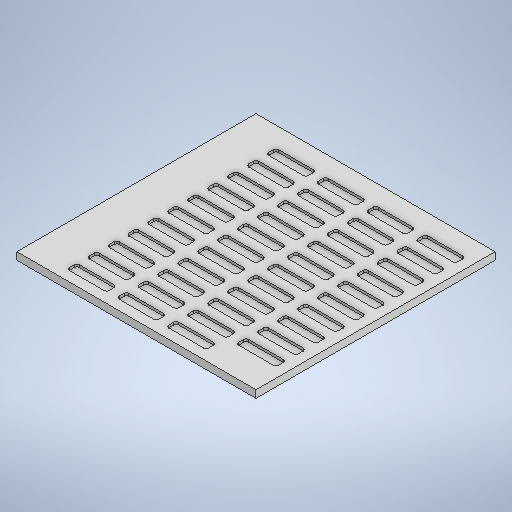
# Autodesk Inventor part: mold plate
Saved by Autodesk Inventor 2025.3 (Build 293356030, 356C)
## iProperties
Created: 2025-07-29
Part Number: mold plate
Material: Generic
Document SubType Name: Modeling
Designer: toppe
Density: 1 g/cm^3
Appearance: Default
Author: toppe
Autodesk Inventor part; units mm, degrees
ref_plane "YZ Plane" through (0, 0, 0) normal (1, 0, 0) x (0, 1, 0)
ref_plane "XZ Plane" through (0, 0, 0) normal (0, 1, 0) x (-1, 0, 0)
ref_plane "XY Plane" through (0, 0, 0) normal (0, 0, 1) x (1, 0, 0)
sketch "Sketch1" plane through (0, 0, 0) normal (0, 1, 0) x (-1, 0, 0)
  line L0 (0, 0) -> (304.8, 0)
  line L1 (304.8, 0) -> (304.8, -304.8)
  line L2 (304.8, -304.8) -> (0, -304.8)
  line L3 (0, -304.8) -> (0, 0)
  dimension "d0" = 304.8
  dimension "d1" = 304.8
  constraints: 8 end point, 2 parallel, 1 horizontal, 1 perpendicular
  measures "d0" distance of L0.end L1.end
  measures "d1" distance of L0.start L0.end
extrude "Extrusion1" add sketch "Sketch1" along normal blind 9.525
sketch "Sketch2" plane through (0, 9.525, 0) normal (0, 1, 0) x (1, 0, 0)
  line L0 (-60.325, 12.7) -> (-15.875, 12.7)
  line L1 (-12.7, 15.875) -> (-12.7, 22.225)
  line L2 (-15.875, 25.4) -> (-60.325, 25.4)
  line L3 (-63.5, 22.225) -> (-63.5, 15.875)
  line L4 (-304.8, 0) -> (0, 0) projected
  line L5 (0, 0) -> (0, 304.8) projected
  arc A0 (-63.5, 15.875) -> (-60.325, 12.7) centre (-60.325, 15.875) ccw
  arc A1 (-60.325, 25.4) -> (-63.5, 22.225) centre (-60.325, 22.225) ccw
  arc A2 (-15.875, 12.7) -> (-12.7, 15.875) centre (-15.875, 15.875) ccw
  arc A3 (-12.7, 22.225) -> (-15.875, 25.4) centre (-15.875, 22.225) ccw
  line L6 (-60.325, 38.1) -> (-15.875, 38.1)
  line L7 (-12.7, 41.275) -> (-12.7, 47.625)
  line L8 (-15.875, 50.8) -> (-60.325, 50.8)
  line L9 (-63.5, 47.625) -> (-63.5, 41.275)
  arc A4 (-15.875, 38.1) -> (-12.7, 41.275) centre (-15.875, 41.275) ccw
  arc A5 (-60.325, 50.8) -> (-63.5, 47.625) centre (-60.325, 47.625) ccw
  arc A6 (-63.5, 41.275) -> (-60.325, 38.1) centre (-60.325, 41.275) ccw
  arc A7 (-12.7, 47.625) -> (-15.875, 50.8) centre (-15.875, 47.625) ccw
  line L10 (-60.325, 63.5) -> (-15.875, 63.5)
  line L11 (-12.7, 66.675) -> (-12.7, 73.025)
  line L12 (-15.875, 76.2) -> (-60.325, 76.2)
  line L13 (-63.5, 73.025) -> (-63.5, 66.675)
  arc A8 (-15.875, 63.5) -> (-12.7, 66.675) centre (-15.875, 66.675) ccw
  arc A9 (-60.325, 76.2) -> (-63.5, 73.025) centre (-60.325, 73.025) ccw
  arc A10 (-63.5, 66.675) -> (-60.325, 63.5) centre (-60.325, 66.675) ccw
  arc A11 (-12.7, 73.025) -> (-15.875, 76.2) centre (-15.875, 73.025) ccw
  line L14 (-60.325, 88.9) -> (-15.875, 88.9)
  line L15 (-12.7, 92.075) -> (-12.7, 98.425)
  line L16 (-15.875, 101.6) -> (-60.325, 101.6)
  line L17 (-63.5, 98.425) -> (-63.5, 92.075)
  arc A12 (-15.875, 88.9) -> (-12.7, 92.075) centre (-15.875, 92.075) ccw
  arc A13 (-60.325, 101.6) -> (-63.5, 98.425) centre (-60.325, 98.425) ccw
  arc A14 (-63.5, 92.075) -> (-60.325, 88.9) centre (-60.325, 92.075) ccw
  arc A15 (-12.7, 98.425) -> (-15.875, 101.6) centre (-15.875, 98.425) ccw
  line L18 (-60.325, 114.3) -> (-15.875, 114.3)
  line L19 (-12.7, 117.475) -> (-12.7, 123.825)
  line L20 (-15.875, 127) -> (-60.325, 127)
  line L21 (-63.5, 123.825) -> (-63.5, 117.475)
  arc A16 (-15.875, 114.3) -> (-12.7, 117.475) centre (-15.875, 117.475) ccw
  arc A17 (-60.325, 127) -> (-63.5, 123.825) centre (-60.325, 123.825) ccw
  arc A18 (-63.5, 117.475) -> (-60.325, 114.3) centre (-60.325, 117.475) ccw
  arc A19 (-12.7, 123.825) -> (-15.875, 127) centre (-15.875, 123.825) ccw
  line L22 (-60.325, 139.7) -> (-15.875, 139.7)
  line L23 (-12.7, 142.875) -> (-12.7, 149.225)
  line L24 (-15.875, 152.4) -> (-60.325, 152.4)
  line L25 (-63.5, 149.225) -> (-63.5, 142.875)
  arc A20 (-15.875, 139.7) -> (-12.7, 142.875) centre (-15.875, 142.875) ccw
  arc A21 (-60.325, 152.4) -> (-63.5, 149.225) centre (-60.325, 149.225) ccw
  arc A22 (-63.5, 142.875) -> (-60.325, 139.7) centre (-60.325, 142.875) ccw
  arc A23 (-12.7, 149.225) -> (-15.875, 152.4) centre (-15.875, 149.225) ccw
  line L26 (-60.325, 165.1) -> (-15.875, 165.1)
  line L27 (-12.7, 168.275) -> (-12.7, 174.625)
  line L28 (-15.875, 177.8) -> (-60.325, 177.8)
  line L29 (-63.5, 174.625) -> (-63.5, 168.275)
  arc A24 (-15.875, 165.1) -> (-12.7, 168.275) centre (-15.875, 168.275) ccw
  arc A25 (-60.325, 177.8) -> (-63.5, 174.625) centre (-60.325, 174.625) ccw
  arc A26 (-63.5, 168.275) -> (-60.325, 165.1) centre (-60.325, 168.275) ccw
  arc A27 (-12.7, 174.625) -> (-15.875, 177.8) centre (-15.875, 174.625) ccw
  line L30 (-60.325, 190.5) -> (-15.875, 190.5)
  line L31 (-12.7, 193.675) -> (-12.7, 200.025)
  line L32 (-15.875, 203.2) -> (-60.325, 203.2)
  line L33 (-63.5, 200.025) -> (-63.5, 193.675)
  arc A28 (-15.875, 190.5) -> (-12.7, 193.675) centre (-15.875, 193.675) ccw
  arc A29 (-60.325, 203.2) -> (-63.5, 200.025) centre (-60.325, 200.025) ccw
  arc A30 (-63.5, 193.675) -> (-60.325, 190.5) centre (-60.325, 193.675) ccw
  arc A31 (-12.7, 200.025) -> (-15.875, 203.2) centre (-15.875, 200.025) ccw
  line L34 (-60.325, 215.9) -> (-15.875, 215.9)
  line L35 (-12.7, 219.075) -> (-12.7, 225.425)
  line L36 (-15.875, 228.6) -> (-60.325, 228.6)
  line L37 (-63.5, 225.425) -> (-63.5, 219.075)
  arc A32 (-15.875, 215.9) -> (-12.7, 219.075) centre (-15.875, 219.075) ccw
  arc A33 (-60.325, 228.6) -> (-63.5, 225.425) centre (-60.325, 225.425) ccw
  arc A34 (-63.5, 219.075) -> (-60.325, 215.9) centre (-60.325, 219.075) ccw
  arc A35 (-12.7, 225.425) -> (-15.875, 228.6) centre (-15.875, 225.425) ccw
  line L38 (-60.325, 241.3) -> (-15.875, 241.3)
  line L39 (-12.7, 244.475) -> (-12.7, 250.825)
  line L40 (-15.875, 254) -> (-60.325, 254)
  line L41 (-63.5, 250.825) -> (-63.5, 244.475)
  arc A36 (-15.875, 241.3) -> (-12.7, 244.475) centre (-15.875, 244.475) ccw
  arc A37 (-60.325, 254) -> (-63.5, 250.825) centre (-60.325, 250.825) ccw
  arc A38 (-63.5, 244.475) -> (-60.325, 241.3) centre (-60.325, 244.475) ccw
  arc A39 (-12.7, 250.825) -> (-15.875, 254) centre (-15.875, 250.825) ccw
  line L42 (-60.325, 266.7) -> (-15.875, 266.7)
  line L43 (-12.7, 269.875) -> (-12.7, 276.225)
  line L44 (-15.875, 279.4) -> (-60.325, 279.4)
  line L45 (-63.5, 276.225) -> (-63.5, 269.875)
  arc A40 (-15.875, 266.7) -> (-12.7, 269.875) centre (-15.875, 269.875) ccw
  arc A41 (-60.325, 279.4) -> (-63.5, 276.225) centre (-60.325, 276.225) ccw
  arc A42 (-63.5, 269.875) -> (-60.325, 266.7) centre (-60.325, 269.875) ccw
  arc A43 (-12.7, 276.225) -> (-15.875, 279.4) centre (-15.875, 276.225) ccw
  line L46 (-123.825, 12.7) -> (-79.375, 12.7)
  line L47 (-76.2, 15.875) -> (-76.2, 22.225)
  line L48 (-79.375, 25.4) -> (-123.825, 25.4)
  line L49 (-127, 22.225) -> (-127, 15.875)
  arc A44 (-79.375, 12.7) -> (-76.2, 15.875) centre (-79.375, 15.875) ccw
  arc A45 (-123.825, 25.4) -> (-127, 22.225) centre (-123.825, 22.225) ccw
  arc A46 (-127, 15.875) -> (-123.825, 12.7) centre (-123.825, 15.875) ccw
  arc A47 (-76.2, 22.225) -> (-79.375, 25.4) centre (-79.375, 22.225) ccw
  line L50 (-123.825, 38.1) -> (-79.375, 38.1)
  line L51 (-76.2, 41.275) -> (-76.2, 47.625)
  line L52 (-79.375, 50.8) -> (-123.825, 50.8)
  line L53 (-127, 47.625) -> (-127, 41.275)
  arc A48 (-79.375, 38.1) -> (-76.2, 41.275) centre (-79.375, 41.275) ccw
  arc A49 (-123.825, 50.8) -> (-127, 47.625) centre (-123.825, 47.625) ccw
  arc A50 (-127, 41.275) -> (-123.825, 38.1) centre (-123.825, 41.275) ccw
  arc A51 (-76.2, 47.625) -> (-79.375, 50.8) centre (-79.375, 47.625) ccw
  line L54 (-123.825, 63.5) -> (-79.375, 63.5)
  line L55 (-76.2, 66.675) -> (-76.2, 73.025)
  line L56 (-79.375, 76.2) -> (-123.825, 76.2)
  line L57 (-127, 73.025) -> (-127, 66.675)
  arc A52 (-79.375, 63.5) -> (-76.2, 66.675) centre (-79.375, 66.675) ccw
  arc A53 (-123.825, 76.2) -> (-127, 73.025) centre (-123.825, 73.025) ccw
  arc A54 (-127, 66.675) -> (-123.825, 63.5) centre (-123.825, 66.675) ccw
  arc A55 (-76.2, 73.025) -> (-79.375, 76.2) centre (-79.375, 73.025) ccw
  line L58 (-123.825, 88.9) -> (-79.375, 88.9)
  line L59 (-76.2, 92.075) -> (-76.2, 98.425)
  line L60 (-79.375, 101.6) -> (-123.825, 101.6)
  line L61 (-127, 98.425) -> (-127, 92.075)
  arc A56 (-79.375, 88.9) -> (-76.2, 92.075) centre (-79.375, 92.075) ccw
  arc A57 (-123.825, 101.6) -> (-127, 98.425) centre (-123.825, 98.425) ccw
  arc A58 (-127, 92.075) -> (-123.825, 88.9) centre (-123.825, 92.075) ccw
  arc A59 (-76.2, 98.425) -> (-79.375, 101.6) centre (-79.375, 98.425) ccw
  line L62 (-123.825, 114.3) -> (-79.375, 114.3)
  line L63 (-76.2, 117.475) -> (-76.2, 123.825)
  line L64 (-79.375, 127) -> (-123.825, 127)
  line L65 (-127, 123.825) -> (-127, 117.475)
  arc A60 (-79.375, 114.3) -> (-76.2, 117.475) centre (-79.375, 117.475) ccw
  arc A61 (-123.825, 127) -> (-127, 123.825) centre (-123.825, 123.825) ccw
  arc A62 (-127, 117.475) -> (-123.825, 114.3) centre (-123.825, 117.475) ccw
  arc A63 (-76.2, 123.825) -> (-79.375, 127) centre (-79.375, 123.825) ccw
  line L66 (-123.825, 139.7) -> (-79.375, 139.7)
  line L67 (-76.2, 142.875) -> (-76.2, 149.225)
  line L68 (-79.375, 152.4) -> (-123.825, 152.4)
  line L69 (-127, 149.225) -> (-127, 142.875)
  arc A64 (-79.375, 139.7) -> (-76.2, 142.875) centre (-79.375, 142.875) ccw
  arc A65 (-123.825, 152.4) -> (-127, 149.225) centre (-123.825, 149.225) ccw
  arc A66 (-127, 142.875) -> (-123.825, 139.7) centre (-123.825, 142.875) ccw
  arc A67 (-76.2, 149.225) -> (-79.375, 152.4) centre (-79.375, 149.225) ccw
  line L70 (-123.825, 165.1) -> (-79.375, 165.1)
  line L71 (-76.2, 168.275) -> (-76.2, 174.625)
  line L72 (-79.375, 177.8) -> (-123.825, 177.8)
  line L73 (-127, 174.625) -> (-127, 168.275)
  arc A68 (-79.375, 165.1) -> (-76.2, 168.275) centre (-79.375, 168.275) ccw
  arc A69 (-123.825, 177.8) -> (-127, 174.625) centre (-123.825, 174.625) ccw
  arc A70 (-127, 168.275) -> (-123.825, 165.1) centre (-123.825, 168.275) ccw
  arc A71 (-76.2, 174.625) -> (-79.375, 177.8) centre (-79.375, 174.625) ccw
  line L74 (-123.825, 190.5) -> (-79.375, 190.5)
  line L75 (-76.2, 193.675) -> (-76.2, 200.025)
  line L76 (-79.375, 203.2) -> (-123.825, 203.2)
  line L77 (-127, 200.025) -> (-127, 193.675)
  arc A72 (-79.375, 190.5) -> (-76.2, 193.675) centre (-79.375, 193.675) ccw
  arc A73 (-123.825, 203.2) -> (-127, 200.025) centre (-123.825, 200.025) ccw
  arc A74 (-127, 193.675) -> (-123.825, 190.5) centre (-123.825, 193.675) ccw
  arc A75 (-76.2, 200.025) -> (-79.375, 203.2) centre (-79.375, 200.025) ccw
  line L78 (-123.825, 215.9) -> (-79.375, 215.9)
  line L79 (-76.2, 219.075) -> (-76.2, 225.425)
  line L80 (-79.375, 228.6) -> (-123.825, 228.6)
  line L81 (-127, 225.425) -> (-127, 219.075)
  arc A76 (-79.375, 215.9) -> (-76.2, 219.075) centre (-79.375, 219.075) ccw
  arc A77 (-123.825, 228.6) -> (-127, 225.425) centre (-123.825, 225.425) ccw
  arc A78 (-127, 219.075) -> (-123.825, 215.9) centre (-123.825, 219.075) ccw
  arc A79 (-76.2, 225.425) -> (-79.375, 228.6) centre (-79.375, 225.425) ccw
  line L82 (-123.825, 241.3) -> (-79.375, 241.3)
  line L83 (-76.2, 244.475) -> (-76.2, 250.825)
  line L84 (-79.375, 254) -> (-123.825, 254)
  line L85 (-127, 250.825) -> (-127, 244.475)
  arc A80 (-79.375, 241.3) -> (-76.2, 244.475) centre (-79.375, 244.475) ccw
  arc A81 (-123.825, 254) -> (-127, 250.825) centre (-123.825, 250.825) ccw
  arc A82 (-127, 244.475) -> (-123.825, 241.3) centre (-123.825, 244.475) ccw
  arc A83 (-76.2, 250.825) -> (-79.375, 254) centre (-79.375, 250.825) ccw
  line L86 (-123.825, 266.7) -> (-79.375, 266.7)
  line L87 (-76.2, 269.875) -> (-76.2, 276.225)
  line L88 (-79.375, 279.4) -> (-123.825, 279.4)
  line L89 (-127, 276.225) -> (-127, 269.875)
  arc A84 (-79.375, 266.7) -> (-76.2, 269.875) centre (-79.375, 269.875) ccw
  arc A85 (-123.825, 279.4) -> (-127, 276.225) centre (-123.825, 276.225) ccw
  arc A86 (-127, 269.875) -> (-123.825, 266.7) centre (-123.825, 269.875) ccw
  arc A87 (-76.2, 276.225) -> (-79.375, 279.4) centre (-79.375, 276.225) ccw
  line L90 (-187.325, 12.7) -> (-142.875, 12.7)
  line L91 (-139.7, 15.875) -> (-139.7, 22.225)
  line L92 (-142.875, 25.4) -> (-187.325, 25.4)
  line L93 (-190.5, 22.225) -> (-190.5, 15.875)
  arc A88 (-142.875, 12.7) -> (-139.7, 15.875) centre (-142.875, 15.875) ccw
  arc A89 (-187.325, 25.4) -> (-190.5, 22.225) centre (-187.325, 22.225) ccw
  arc A90 (-190.5, 15.875) -> (-187.325, 12.7) centre (-187.325, 15.875) ccw
  arc A91 (-139.7, 22.225) -> (-142.875, 25.4) centre (-142.875, 22.225) ccw
  line L94 (-187.325, 38.1) -> (-142.875, 38.1)
  line L95 (-139.7, 41.275) -> (-139.7, 47.625)
  line L96 (-142.875, 50.8) -> (-187.325, 50.8)
  line L97 (-190.5, 47.625) -> (-190.5, 41.275)
  arc A92 (-142.875, 38.1) -> (-139.7, 41.275) centre (-142.875, 41.275) ccw
  arc A93 (-187.325, 50.8) -> (-190.5, 47.625) centre (-187.325, 47.625) ccw
  arc A94 (-190.5, 41.275) -> (-187.325, 38.1) centre (-187.325, 41.275) ccw
  arc A95 (-139.7, 47.625) -> (-142.875, 50.8) centre (-142.875, 47.625) ccw
  line L98 (-187.325, 63.5) -> (-142.875, 63.5)
  line L99 (-139.7, 66.675) -> (-139.7, 73.025)
  line L100 (-142.875, 76.2) -> (-187.325, 76.2)
  line L101 (-190.5, 73.025) -> (-190.5, 66.675)
  arc A96 (-142.875, 63.5) -> (-139.7, 66.675) centre (-142.875, 66.675) ccw
  arc A97 (-187.325, 76.2) -> (-190.5, 73.025) centre (-187.325, 73.025) ccw
  arc A98 (-190.5, 66.675) -> (-187.325, 63.5) centre (-187.325, 66.675) ccw
  arc A99 (-139.7, 73.025) -> (-142.875, 76.2) centre (-142.875, 73.025) ccw
  line L102 (-187.325, 88.9) -> (-142.875, 88.9)
  line L103 (-139.7, 92.075) -> (-139.7, 98.425)
  line L104 (-142.875, 101.6) -> (-187.325, 101.6)
  line L105 (-190.5, 98.425) -> (-190.5, 92.075)
  arc A100 (-142.875, 88.9) -> (-139.7, 92.075) centre (-142.875, 92.075) ccw
  arc A101 (-187.325, 101.6) -> (-190.5, 98.425) centre (-187.325, 98.425) ccw
  arc A102 (-190.5, 92.075) -> (-187.325, 88.9) centre (-187.325, 92.075) ccw
  arc A103 (-139.7, 98.425) -> (-142.875, 101.6) centre (-142.875, 98.425) ccw
  line L106 (-187.325, 114.3) -> (-142.875, 114.3)
  line L107 (-139.7, 117.475) -> (-139.7, 123.825)
  line L108 (-142.875, 127) -> (-187.325, 127)
  line L109 (-190.5, 123.825) -> (-190.5, 117.475)
  arc A104 (-142.875, 114.3) -> (-139.7, 117.475) centre (-142.875, 117.475) ccw
  arc A105 (-187.325, 127) -> (-190.5, 123.825) centre (-187.325, 123.825) ccw
  arc A106 (-190.5, 117.475) -> (-187.325, 114.3) centre (-187.325, 117.475) ccw
  arc A107 (-139.7, 123.825) -> (-142.875, 127) centre (-142.875, 123.825) ccw
  line L110 (-187.325, 139.7) -> (-142.875, 139.7)
  line L111 (-139.7, 142.875) -> (-139.7, 149.225)
  line L112 (-142.875, 152.4) -> (-187.325, 152.4)
  line L113 (-190.5, 149.225) -> (-190.5, 142.875)
  arc A108 (-142.875, 139.7) -> (-139.7, 142.875) centre (-142.875, 142.875) ccw
  arc A109 (-187.325, 152.4) -> (-190.5, 149.225) centre (-187.325, 149.225) ccw
  arc A110 (-190.5, 142.875) -> (-187.325, 139.7) centre (-187.325, 142.875) ccw
  arc A111 (-139.7, 149.225) -> (-142.875, 152.4) centre (-142.875, 149.225) ccw
  line L114 (-187.325, 165.1) -> (-142.875, 165.1)
  line L115 (-139.7, 168.275) -> (-139.7, 174.625)
  line L116 (-142.875, 177.8) -> (-187.325, 177.8)
  line L117 (-190.5, 174.625) -> (-190.5, 168.275)
  arc A112 (-142.875, 165.1) -> (-139.7, 168.275) centre (-142.875, 168.275) ccw
  arc A113 (-187.325, 177.8) -> (-190.5, 174.625) centre (-187.325, 174.625) ccw
  arc A114 (-190.5, 168.275) -> (-187.325, 165.1) centre (-187.325, 168.275) ccw
  arc A115 (-139.7, 174.625) -> (-142.875, 177.8) centre (-142.875, 174.625) ccw
  line L118 (-187.325, 190.5) -> (-142.875, 190.5)
  line L119 (-139.7, 193.675) -> (-139.7, 200.025)
  line L120 (-142.875, 203.2) -> (-187.325, 203.2)
  line L121 (-190.5, 200.025) -> (-190.5, 193.675)
  arc A116 (-142.875, 190.5) -> (-139.7, 193.675) centre (-142.875, 193.675) ccw
  arc A117 (-187.325, 203.2) -> (-190.5, 200.025) centre (-187.325, 200.025) ccw
  arc A118 (-190.5, 193.675) -> (-187.325, 190.5) centre (-187.325, 193.675) ccw
  arc A119 (-139.7, 200.025) -> (-142.875, 203.2) centre (-142.875, 200.025) ccw
  line L122 (-187.325, 215.9) -> (-142.875, 215.9)
  line L123 (-139.7, 219.075) -> (-139.7, 225.425)
  line L124 (-142.875, 228.6) -> (-187.325, 228.6)
  line L125 (-190.5, 225.425) -> (-190.5, 219.075)
  arc A120 (-142.875, 215.9) -> (-139.7, 219.075) centre (-142.875, 219.075) ccw
  arc A121 (-187.325, 228.6) -> (-190.5, 225.425) centre (-187.325, 225.425) ccw
  arc A122 (-190.5, 219.075) -> (-187.325, 215.9) centre (-187.325, 219.075) ccw
  arc A123 (-139.7, 225.425) -> (-142.875, 228.6) centre (-142.875, 225.425) ccw
  line L126 (-187.325, 241.3) -> (-142.875, 241.3)
  line L127 (-139.7, 244.475) -> (-139.7, 250.825)
  line L128 (-142.875, 254) -> (-187.325, 254)
  line L129 (-190.5, 250.825) -> (-190.5, 244.475)
  arc A124 (-142.875, 241.3) -> (-139.7, 244.475) centre (-142.875, 244.475) ccw
  arc A125 (-187.325, 254) -> (-190.5, 250.825) centre (-187.325, 250.825) ccw
  arc A126 (-190.5, 244.475) -> (-187.325, 241.3) centre (-187.325, 244.475) ccw
  arc A127 (-139.7, 250.825) -> (-142.875, 254) centre (-142.875, 250.825) ccw
  line L130 (-187.325, 266.7) -> (-142.875, 266.7)
  line L131 (-139.7, 269.875) -> (-139.7, 276.225)
  line L132 (-142.875, 279.4) -> (-187.325, 279.4)
  line L133 (-190.5, 276.225) -> (-190.5, 269.875)
  arc A128 (-142.875, 266.7) -> (-139.7, 269.875) centre (-142.875, 269.875) ccw
  arc A129 (-187.325, 279.4) -> (-190.5, 276.225) centre (-187.325, 276.225) ccw
  arc A130 (-190.5, 269.875) -> (-187.325, 266.7) centre (-187.325, 269.875) ccw
  arc A131 (-139.7, 276.225) -> (-142.875, 279.4) centre (-142.875, 276.225) ccw
  line L134 (-250.825, 12.7) -> (-206.375, 12.7)
  line L135 (-203.2, 15.875) -> (-203.2, 22.225)
  line L136 (-206.375, 25.4) -> (-250.825, 25.4)
  line L137 (-254, 22.225) -> (-254, 15.875)
  arc A132 (-206.375, 12.7) -> (-203.2, 15.875) centre (-206.375, 15.875) ccw
  arc A133 (-250.825, 25.4) -> (-254, 22.225) centre (-250.825, 22.225) ccw
  arc A134 (-254, 15.875) -> (-250.825, 12.7) centre (-250.825, 15.875) ccw
  arc A135 (-203.2, 22.225) -> (-206.375, 25.4) centre (-206.375, 22.225) ccw
  line L138 (-250.825, 38.1) -> (-206.375, 38.1)
  line L139 (-203.2, 41.275) -> (-203.2, 47.625)
  line L140 (-206.375, 50.8) -> (-250.825, 50.8)
  line L141 (-254, 47.625) -> (-254, 41.275)
  arc A136 (-206.375, 38.1) -> (-203.2, 41.275) centre (-206.375, 41.275) ccw
  arc A137 (-250.825, 50.8) -> (-254, 47.625) centre (-250.825, 47.625) ccw
  arc A138 (-254, 41.275) -> (-250.825, 38.1) centre (-250.825, 41.275) ccw
  arc A139 (-203.2, 47.625) -> (-206.375, 50.8) centre (-206.375, 47.625) ccw
  line L142 (-250.825, 63.5) -> (-206.375, 63.5)
  line L143 (-203.2, 66.675) -> (-203.2, 73.025)
  line L144 (-206.375, 76.2) -> (-250.825, 76.2)
  line L145 (-254, 73.025) -> (-254, 66.675)
  arc A140 (-206.375, 63.5) -> (-203.2, 66.675) centre (-206.375, 66.675) ccw
  arc A141 (-250.825, 76.2) -> (-254, 73.025) centre (-250.825, 73.025) ccw
  arc A142 (-254, 66.675) -> (-250.825, 63.5) centre (-250.825, 66.675) ccw
  arc A143 (-203.2, 73.025) -> (-206.375, 76.2) centre (-206.375, 73.025) ccw
  line L146 (-250.825, 88.9) -> (-206.375, 88.9)
  line L147 (-203.2, 92.075) -> (-203.2, 98.425)
  line L148 (-206.375, 101.6) -> (-250.825, 101.6)
  line L149 (-254, 98.425) -> (-254, 92.075)
  arc A144 (-206.375, 88.9) -> (-203.2, 92.075) centre (-206.375, 92.075) ccw
  arc A145 (-250.825, 101.6) -> (-254, 98.425) centre (-250.825, 98.425) ccw
  arc A146 (-254, 92.075) -> (-250.825, 88.9) centre (-250.825, 92.075) ccw
  arc A147 (-203.2, 98.425) -> (-206.375, 101.6) centre (-206.375, 98.425) ccw
  line L150 (-250.825, 114.3) -> (-206.375, 114.3)
  line L151 (-203.2, 117.475) -> (-203.2, 123.825)
  line L152 (-206.375, 127) -> (-250.825, 127)
  line L153 (-254, 123.825) -> (-254, 117.475)
  arc A148 (-206.375, 114.3) -> (-203.2, 117.475) centre (-206.375, 117.475) ccw
  arc A149 (-250.825, 127) -> (-254, 123.825) centre (-250.825, 123.825) ccw
  arc A150 (-254, 117.475) -> (-250.825, 114.3) centre (-250.825, 117.475) ccw
  arc A151 (-203.2, 123.825) -> (-206.375, 127) centre (-206.375, 123.825) ccw
  line L154 (-250.825, 139.7) -> (-206.375, 139.7)
  line L155 (-203.2, 142.875) -> (-203.2, 149.225)
  line L156 (-206.375, 152.4) -> (-250.825, 152.4)
  line L157 (-254, 149.225) -> (-254, 142.875)
  arc A152 (-206.375, 139.7) -> (-203.2, 142.875) centre (-206.375, 142.875) ccw
  arc A153 (-250.825, 152.4) -> (-254, 149.225) centre (-250.825, 149.225) ccw
  arc A154 (-254, 142.875) -> (-250.825, 139.7) centre (-250.825, 142.875) ccw
  arc A155 (-203.2, 149.225) -> (-206.375, 152.4) centre (-206.375, 149.225) ccw
  line L158 (-250.825, 165.1) -> (-206.375, 165.1)
  line L159 (-203.2, 168.275) -> (-203.2, 174.625)
  line L160 (-206.375, 177.8) -> (-250.825, 177.8)
  line L161 (-254, 174.625) -> (-254, 168.275)
  arc A156 (-206.375, 165.1) -> (-203.2, 168.275) centre (-206.375, 168.275) ccw
  arc A157 (-250.825, 177.8) -> (-254, 174.625) centre (-250.825, 174.625) ccw
  arc A158 (-254, 168.275) -> (-250.825, 165.1) centre (-250.825, 168.275) ccw
  arc A159 (-203.2, 174.625) -> (-206.375, 177.8) centre (-206.375, 174.625) ccw
  line L162 (-250.825, 190.5) -> (-206.375, 190.5)
  line L163 (-203.2, 193.675) -> (-203.2, 200.025)
  line L164 (-206.375, 203.2) -> (-250.825, 203.2)
  line L165 (-254, 200.025) -> (-254, 193.675)
  arc A160 (-206.375, 190.5) -> (-203.2, 193.675) centre (-206.375, 193.675) ccw
  arc A161 (-250.825, 203.2) -> (-254, 200.025) centre (-250.825, 200.025) ccw
  arc A162 (-254, 193.675) -> (-250.825, 190.5) centre (-250.825, 193.675) ccw
  arc A163 (-203.2, 200.025) -> (-206.375, 203.2) centre (-206.375, 200.025) ccw
  line L166 (-250.825, 215.9) -> (-206.375, 215.9)
  line L167 (-203.2, 219.075) -> (-203.2, 225.425)
  line L168 (-206.375, 228.6) -> (-250.825, 228.6)
  line L169 (-254, 225.425) -> (-254, 219.075)
  arc A164 (-206.375, 215.9) -> (-203.2, 219.075) centre (-206.375, 219.075) ccw
  arc A165 (-250.825, 228.6) -> (-254, 225.425) centre (-250.825, 225.425) ccw
  arc A166 (-254, 219.075) -> (-250.825, 215.9) centre (-250.825, 219.075) ccw
  arc A167 (-203.2, 225.425) -> (-206.375, 228.6) centre (-206.375, 225.425) ccw
  line L170 (-250.825, 241.3) -> (-206.375, 241.3)
  line L171 (-203.2, 244.475) -> (-203.2, 250.825)
  line L172 (-206.375, 254) -> (-250.825, 254)
  line L173 (-254, 250.825) -> (-254, 244.475)
  arc A168 (-206.375, 241.3) -> (-203.2, 244.475) centre (-206.375, 244.475) ccw
  arc A169 (-250.825, 254) -> (-254, 250.825) centre (-250.825, 250.825) ccw
  arc A170 (-254, 244.475) -> (-250.825, 241.3) centre (-250.825, 244.475) ccw
  arc A171 (-203.2, 250.825) -> (-206.375, 254) centre (-206.375, 250.825) ccw
  line L174 (-250.825, 266.7) -> (-206.375, 266.7)
  line L175 (-203.2, 269.875) -> (-203.2, 276.225)
  line L176 (-206.375, 279.4) -> (-250.825, 279.4)
  line L177 (-254, 276.225) -> (-254, 269.875)
  arc A172 (-206.375, 266.7) -> (-203.2, 269.875) centre (-206.375, 269.875) ccw
  arc A173 (-250.825, 279.4) -> (-254, 276.225) centre (-250.825, 276.225) ccw
  arc A174 (-254, 269.875) -> (-250.825, 266.7) centre (-250.825, 269.875) ccw
  arc A175 (-203.2, 276.225) -> (-206.375, 279.4) centre (-206.375, 276.225) ccw
  point P0 (-63.5, 12.7)
  point P1 (-12.7, 25.4)
  point P2 (-63.5, 25.4)
  point P3 (-12.7, 19.05)
  point P4 (0, 25.4)
  point P5 (-63.5, 38.1)
  point P6 (-12.7, 50.8)
  point P7 (-12.7, 44.45)
  point P8 (-63.5, 50.8)
  point P9 (0, 50.8)
  point P10 (-63.5, 63.5)
  point P11 (-12.7, 76.2)
  point P12 (-12.7, 69.85)
  point P13 (-63.5, 76.2)
  point P14 (0, 76.2)
  point P15 (-63.5, 88.9)
  point P16 (-12.7, 101.6)
  point P17 (-12.7, 95.25)
  point P18 (-63.5, 101.6)
  point P19 (0, 101.6)
  point P20 (-63.5, 114.3)
  point P21 (-12.7, 127)
  point P22 (-12.7, 120.65)
  point P23 (-63.5, 127)
  point P24 (0, 127)
  point P25 (-63.5, 139.7)
  point P26 (-12.7, 152.4)
  point P27 (-12.7, 146.05)
  point P28 (-63.5, 152.4)
  point P29 (0, 152.4)
  point P30 (-63.5, 165.1)
  point P31 (-12.7, 177.8)
  point P32 (-12.7, 171.45)
  point P33 (-63.5, 177.8)
  point P34 (0, 177.8)
  point P35 (-63.5, 190.5)
  point P36 (-12.7, 203.2)
  point P37 (-12.7, 196.85)
  point P38 (-63.5, 203.2)
  point P39 (0, 203.2)
  point P40 (-63.5, 215.9)
  point P41 (-12.7, 228.6)
  point P42 (-12.7, 222.25)
  point P43 (-63.5, 228.6)
  point P44 (0, 228.6)
  point P45 (-63.5, 241.3)
  point P46 (-12.7, 254)
  point P47 (-12.7, 247.65)
  point P48 (-63.5, 254)
  point P49 (0, 254)
  point P50 (-63.5, 266.7)
  point P51 (-12.7, 279.4)
  point P52 (-12.7, 273.05)
  point P53 (-63.5, 279.4)
  point P54 (-63.5, 0)
  point P55 (-127, 12.7)
  point P56 (-76.2, 25.4)
  point P57 (-76.2, 19.05)
  point P58 (-127, 25.4)
  point P59 (-63.5, 25.4)
  point P60 (-127, 38.1)
  point P61 (-76.2, 50.8)
  point P62 (-76.2, 44.45)
  point P63 (-127, 50.8)
  point P64 (-63.5, 50.8)
  point P65 (-127, 63.5)
  point P66 (-76.2, 76.2)
  point P67 (-76.2, 69.85)
  point P68 (-127, 76.2)
  point P69 (-63.5, 76.2)
  point P70 (-127, 88.9)
  point P71 (-76.2, 101.6)
  point P72 (-76.2, 95.25)
  point P73 (-127, 101.6)
  point P74 (-63.5, 101.6)
  point P75 (-127, 114.3)
  point P76 (-76.2, 127)
  point P77 (-76.2, 120.65)
  point P78 (-127, 127)
  point P79 (-63.5, 127)
  point P80 (-127, 139.7)
  point P81 (-76.2, 152.4)
  point P82 (-76.2, 146.05)
  point P83 (-127, 152.4)
  point P84 (-63.5, 152.4)
  point P85 (-127, 165.1)
  point P86 (-76.2, 177.8)
  point P87 (-76.2, 171.45)
  point P88 (-127, 177.8)
  point P89 (-63.5, 177.8)
  point P90 (-127, 190.5)
  point P91 (-76.2, 203.2)
  point P92 (-76.2, 196.85)
  point P93 (-127, 203.2)
  point P94 (-63.5, 203.2)
  point P95 (-127, 215.9)
  point P96 (-76.2, 228.6)
  point P97 (-76.2, 222.25)
  point P98 (-127, 228.6)
  point P99 (-63.5, 228.6)
  point P100 (-127, 241.3)
  point P101 (-76.2, 254)
  point P102 (-76.2, 247.65)
  point P103 (-127, 254)
  point P104 (-63.5, 254)
  point P105 (-127, 266.7)
  point P106 (-76.2, 279.4)
  point P107 (-76.2, 273.05)
  point P108 (-127, 279.4)
  point P109 (-127, 0)
  point P110 (-190.5, 12.7)
  point P111 (-139.7, 25.4)
  point P112 (-139.7, 19.05)
  point P113 (-190.5, 25.4)
  point P114 (-127, 25.4)
  point P115 (-190.5, 38.1)
  point P116 (-139.7, 50.8)
  point P117 (-139.7, 44.45)
  point P118 (-190.5, 50.8)
  point P119 (-127, 50.8)
  point P120 (-190.5, 63.5)
  point P121 (-139.7, 76.2)
  point P122 (-139.7, 69.85)
  point P123 (-190.5, 76.2)
  point P124 (-127, 76.2)
  point P125 (-190.5, 88.9)
  point P126 (-139.7, 101.6)
  point P127 (-139.7, 95.25)
  point P128 (-190.5, 101.6)
  point P129 (-127, 101.6)
  point P130 (-190.5, 114.3)
  point P131 (-139.7, 127)
  point P132 (-139.7, 120.65)
  point P133 (-190.5, 127)
  point P134 (-127, 127)
  point P135 (-190.5, 139.7)
  point P136 (-139.7, 152.4)
  point P137 (-139.7, 146.05)
  point P138 (-190.5, 152.4)
  point P139 (-127, 152.4)
  point P140 (-190.5, 165.1)
  point P141 (-139.7, 177.8)
  point P142 (-139.7, 171.45)
  point P143 (-190.5, 177.8)
  point P144 (-127, 177.8)
  point P145 (-190.5, 190.5)
  point P146 (-139.7, 203.2)
  point P147 (-139.7, 196.85)
  point P148 (-190.5, 203.2)
  point P149 (-127, 203.2)
  point P150 (-190.5, 215.9)
  point P151 (-139.7, 228.6)
  point P152 (-139.7, 222.25)
  point P153 (-190.5, 228.6)
  point P154 (-127, 228.6)
  point P155 (-190.5, 241.3)
  point P156 (-139.7, 254)
  point P157 (-139.7, 247.65)
  point P158 (-190.5, 254)
  point P159 (-127, 254)
  point P160 (-190.5, 266.7)
  point P161 (-139.7, 279.4)
  point P162 (-139.7, 273.05)
  point P163 (-190.5, 279.4)
  point P164 (-190.5, 0)
  point P165 (-254, 12.7)
  point P166 (-203.2, 25.4)
  point P167 (-203.2, 19.05)
  point P168 (-254, 25.4)
  point P169 (-190.5, 25.4)
  point P170 (-254, 38.1)
  point P171 (-203.2, 50.8)
  point P172 (-203.2, 44.45)
  point P173 (-254, 50.8)
  point P174 (-190.5, 50.8)
  point P175 (-254, 63.5)
  point P176 (-203.2, 76.2)
  point P177 (-203.2, 69.85)
  point P178 (-254, 76.2)
  point P179 (-190.5, 76.2)
  point P180 (-254, 88.9)
  point P181 (-203.2, 101.6)
  point P182 (-203.2, 95.25)
  point P183 (-254, 101.6)
  point P184 (-190.5, 101.6)
  point P185 (-254, 114.3)
  point P186 (-203.2, 127)
  point P187 (-203.2, 120.65)
  point P188 (-254, 127)
  point P189 (-190.5, 127)
  point P190 (-254, 139.7)
  point P191 (-203.2, 152.4)
  point P192 (-203.2, 146.05)
  point P193 (-254, 152.4)
  point P194 (-190.5, 152.4)
  point P195 (-254, 165.1)
  point P196 (-203.2, 177.8)
  point P197 (-203.2, 171.45)
  point P198 (-254, 177.8)
  point P199 (-190.5, 177.8)
  dimension "d4" = 50.8
  dimension "d5" = 12.7
  dimension "d6" = 12.7
  dimension "d7" = 12.7
  dimension "d8" = 3.175
  dimension "d13" = 25.4
  dimension "d16" = 63.5
  constraints: 352 end point, 352 point on circle, 264 point on line, 176 centre point, 8 tangent, 3 equal radius, 2 horizontal, 2 parallel, 1 midpoint, 1 perpendicular, 1 vertical, 1075 other
  measures "d4" distance of point (-12.7, 25.4) point (-63.5, 25.4)
  measures "d5" distance of point (-63.5, 25.4) point (-63.5, 12.7)
  measures "d6" distance between parallel lines of L4 L0
  measures "d7" distance from line of L5 point (-12.7, 19.05)
  measures "d8" radius of A0
  measures "d13" distance of L4.end point (0, 25.4)
  measures "d16" distance of L4.end point (-63.5, 0)
extrude "Extrusion2" cut sketch "Sketch2" against normal blind 3.175 contours A6 L9 A5 L8 A7 L7 A4 L6 | A10 L13 A9 L12 A11 L11 A8 L10 | A14 L17 A13 L16 A15 L15 A12 L14 | A18 L21 A17 L20 A19 L19 A16 L18 | A22 L25 A21 L24 A23 L23 A20 L22 | A26 L29 A25 L28 A27 L27 A24 L26 | A30 L33 A29 L32 A31 L31 A28 L30 | A34 L37 A33 L36 A35 L35 A32 L34 | A38 L41 A37 L40 A39 L39 A36 L38 | A42 L45 A41 L44 A43 L43 A40 L42 | A46 L49 A45 L48 A47 L47 A44 L46 | A50 L53 A49 L52 A51 L51 A48 L50 | A54 L57 A53 L56 A55 L55 A52 L54 | A58 L61 A57 L60 A59 L59 A56 L58 | A62 L65 A61 L64 A63 L63 A60 L62 | A66 L69 A65 L68 A67 L67 A64 L66 | A70 L73 A69 L72 A71 L71 A68 L70 | A74 L77 A73 L76 A75 L75 A72 L74 | A78 L81 A77 L80 A79 L79 A76 L78 | A82 L85 A81 L84 A83 L83 A80 L82 | A86 L89 A85 L88 A87 L87 A84 L86 | A90 L93 A89 L92 A91 L91 A88 L90 | A94 L97 A93 L96 A95 L95 A92 L94 | A98 L101 A97 L100 A99 L99 A96 L98 | A102 L105 A101 L104 A103 L103 A100 L102 | A106 L109 A105 L108 A107 L107 A104 L106 | A110 L113 A109 L112 A111 L111 A108 L110 | A114 L117 A113 L116 A115 L115 A112 L114 | A118 L121 A117 L120 A119 L119 A116 L118 | A122 L125 A121 L124 A123 L123 A120 L122 | A126 L129 A125 L128 A127 L127 A124 L126 | A130 L133 A129 L132 A131 L131 A128 L130 | A134 L137 A133 L136 A135 L135 A132 L134 | A138 L141 A137 L140 A139 L139 A136 L138 | A142 L145 A141 L144 A143 L143 A140 L142 | A146 L149 A145 L148 A147 L147 A144 L146 | A150 L153 A149 L152 A151 L151 A148 L150 | A154 L157 A153 L156 A155 L155 A152 L154 | A158 L161 A157 L160 A159 L159 A156 L158 | A162 L165 A161 L164 A163 L163 A160 L162 | A166 L169 A165 L168 A167 L167 A164 L166 | A170 L173 A169 L172 A171 L171 A168 L170 | A174 L177 A173 L176 A175 L175 A172 L174
body "Solid1"
